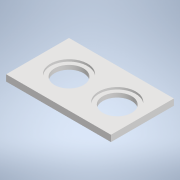
# Autodesk Inventor part: Proto_Valve_Fitting_TestPlate
Saved by Autodesk Inventor 2022.2 (Build 262287000, 287)
## iProperties
Created: 2022-01-18
Part Number: Proto_Valve_Fitting_TestPlate
Material: Generic
Document SubType Name: Modeling
Designer: siwat
Density: 1 g/cm^3
Appearance: Default
Author: siwat
Autodesk Inventor part; units mm, degrees
ref_plane "YZ Plane" through (0, 0, 0) normal (1, 0, 0) x (0, 1, 0)
ref_plane "XZ Plane" through (0, 0, 0) normal (0, 1, 0) x (-1, 0, 0)
ref_plane "XY Plane" through (0, 0, 0) normal (0, 0, 1) x (1, 0, 0)
sketch "Sketch1" plane through (0, 0, 0) normal (0, 1, 0) x (-1, 0, 0)
  line L0 (0, 0) -> (-50, 0)
  line L1 (-50, 0) -> (-50, -30)
  line L2 (-50, -30) -> (0, -30)
  line L3 (0, -30) -> (0, 0)
  dimension "d0" = 50
  dimension "d1" = 30
  constraints: 8 end point, 2 parallel, 1 coincident, 1 horizontal, 1 perpendicular
  measures "d0" distance of L2.end L1.end
  measures "d1" distance of L1.end L0.end
extrude "Extrusion1" add sketch "Sketch1" along normal blind 3
sketch "Sketch2" plane through (0, 3, 0) normal (0, 1, 0) x (1, 0, 0)
  circle A0 centre (15, 15) radius 8.8
  line L0 (0, 30) -> (0, 0) projected
  line L1 (0, 0) -> (50, 0) projected
  circle A1 centre (38, 15) radius 8.8
  dimension "d4" = 17.6
  dimension "d5" = 15
  dimension "d6" = 15
  dimension "d12" = 17.6
  dimension "d16" = 0
  dimension "d17" = 23
  constraints: 2 centre point
  measures "d4" diameter of A0
  measures "d5" distance from line of A0.centre L0
  measures "d6" distance from line of L1 A0.centre
  measures "d12" diameter of A1
  measures "d16" vertical distance of A0.centre A1.centre
  measures "d17" distance of A1.centre A0.centre
extrude "Extrusion2" cut sketch "Sketch2" against normal blind 1
sketch "Sketch3" plane through (15, 2, -15) normal (0, 1, 0) x (1, 0, 0)
  circle A0 centre (0, 0) radius 6.9
  circle A1 centre (23, 0) radius 6.9
  circle A2 centre (23, 0) radius 8.8 projected
  point P0 (-15, -15)
  point P1 (-13.4125, -13.4125)
  dimension "d9" = 13.8
  dimension "d13" = 13.8
  dimension "d14" = 0
  dimension "d15" = 0
  constraints: 2 centre point
  measures "d9" diameter of A0
  measures "d13" diameter of A1
  measures "d14" distance of A2.centre A1.centre
  measures "d15" distance of A2.centre A1.centre
extrude "Extrusion3" cut sketch "Sketch3" against normal through all contours A0 | A1
body "Solid1"
